Autodesk Fusion 360 part; units mm, degrees
note: some values were not read from the file. Set by a fixed rule: which sketch regions a step uses.
(part 14 of 59)
  spline S77 degree 5 poles (17.8091, 35.4448) (17.8092, 35.4448) (17.8093, 35.445) (17.8095, 35.4453) (17.8098, 35.4457) (17.8103, 35.4463) (17.8108, 35.4469) (17.8114, 35.4477) (17.812, 35.4486) (17.8127, 35.4496) (17.8135, 35.4506) (17.8144, 35.4518) (17.8153, 35.453) (17.8162, 35.4543) (17.8172, 35.4557) (17.8183, 35.4572) (17.8195, 35.4588) (17.8207, 35.4604) (17.8219, 35.4622) (17.8232, 35.464) (17.8246, 35.4659) (17.826, 35.4679) (17.8274, 35.4699) (17.8289, 35.4721) (17.8305, 35.4743) (17.8321, 35.4766) (17.8337, 35.479) (17.8354, 35.4814) (17.8372, 35.484) (17.8389, 35.4866) (17.8408, 35.4893) (17.8427, 35.492) (17.8446, 35.4948) (17.8465, 35.4978) (17.8485, 35.5007) (17.8506, 35.5038) (17.8527, 35.5069) (17.8548, 35.5101) (17.857, 35.5134) (17.8592, 35.5167) (17.8614, 35.5201) (17.8637, 35.5236) (17.866, 35.5271) (17.8683, 35.5308) (17.8707, 35.5344) (17.8731, 35.5382) (17.8756, 35.542) (17.8781, 35.5459) (17.8806, 35.5499) (17.8831, 35.5539) (17.8857, 35.558) (17.8883, 35.5621) (17.891, 35.5664) (17.8937, 35.5706) (17.8964, 35.575) (17.8991, 35.5794) (17.9019, 35.5839) (17.9047, 35.5884) (17.9075, 35.593) (17.9103, 35.5977) (17.9132, 35.6024) (17.9161, 35.6072) (17.9191, 35.6121) (17.922, 35.617) (17.925, 35.622) (17.928, 35.627) (17.931, 35.6321) (17.9341, 35.6373) (17.9372, 35.6425) (17.9403, 35.6478) (17.9434, 35.6531) (17.9466, 35.6585) (17.9497, 35.664) (17.9529, 35.6695) (17.9562, 35.6751) (17.9594, 35.6807) (17.9627, 35.6864) (17.9659, 35.6921) (17.9692, 35.6979) (17.9726, 35.7038) (17.9759, 35.7097) (17.9793, 35.7157) (17.9826, 35.7217) (17.986, 35.7278) (17.9895, 35.734) (17.9929, 35.7402) (17.9963, 35.7464) (17.9998, 35.7527) (18.0033, 35.7591) (18.0068, 35.7655) (18.0103, 35.772) (18.0139, 35.7785) (18.0174, 35.7851) (18.021, 35.7918) (18.0246, 35.7984) (18.0282, 35.8052) (18.0318, 35.812) (18.0354, 35.8188) (18.039, 35.8257) (18.0427, 35.8327) (18.0464, 35.8397) (18.0501, 35.8468) (18.0538, 35.8539) (18.0575, 35.861) (18.0612, 35.8683) (18.0649, 35.8755) (18.0687, 35.8828) (18.0724, 35.8902) (18.0762, 35.8976) (18.08, 35.9051) (18.0838, 35.9126) (18.0876, 35.9202) (18.0914, 35.9278) (18.0952, 35.9355) (18.0991, 35.9432) (18.1029, 35.951) (18.1068, 35.9588) (18.1106, 35.9666) (18.1145, 35.9746) (18.1184, 35.9825) (18.1223, 35.9905) (18.1262, 35.9986) (18.1301, 36.0067) (18.134, 36.0149) (18.1379, 36.0231) (18.1419, 36.0313) (18.1458, 36.0396) (18.1498, 36.048) (18.1537, 36.0564) (18.1577, 36.0648) (18.1617, 36.0733) (18.1657, 36.0818) (18.1696, 36.0904) (18.1736, 36.0991) (18.1776, 36.1077) (18.1816, 36.1165) (18.1857, 36.1252) (18.1897, 36.134) (18.1937, 36.1429) (18.1977, 36.1518) (18.2018, 36.1607) (18.2058, 36.1697) (18.2098, 36.1788) (18.2139, 36.1879) (18.2179, 36.197) (18.222, 36.2062) (18.226, 36.2154) (18.2301, 36.2247) (18.2342, 36.234) (18.2383, 36.2433) (18.2423, 36.2527) (18.2464, 36.2622) (18.2505, 36.2716) (18.2546, 36.2812) (18.2587, 36.2907) (18.2627, 36.3004) (18.2668, 36.31) (18.2709, 36.3197) (18.275, 36.3295) (18.2791, 36.3393) (18.2832, 36.3491) (18.2873, 36.359) (18.2914, 36.3689) (18.2955, 36.3788) (18.2996, 36.3888) (18.3038, 36.3989) (18.3079, 36.409) (18.312, 36.4191) (18.3161, 36.4292) (18.3202, 36.4395) (18.3243, 36.4497) (18.3284, 36.46) (18.3325, 36.4703) (18.3366, 36.4807) (18.3408, 36.4911) (18.3449, 36.5016) (18.349, 36.5121) (18.3531, 36.5226) (18.3572, 36.5332) (18.3613, 36.5438) (18.3654, 36.5545) (18.3695, 36.5652) (18.3736, 36.5759) (18.3777, 36.5867) (18.3818, 36.5975) (18.3859, 36.6084) (18.39, 36.6193) (18.3941, 36.6302) (18.3982, 36.6412) (18.4023, 36.6522) (18.4064, 36.6633) (18.4105, 36.6744) (18.4146, 36.6855) (18.4187, 36.6967) (18.4228, 36.7079) (18.4269, 36.7191) (18.4309, 36.7304) (18.435, 36.7417) (18.4391, 36.7531) (18.4431, 36.7645) (18.4472, 36.776) (18.4513, 36.7874) (18.4553, 36.799) (18.4594, 36.8105) (18.4634, 36.8221) (18.4675, 36.8337) (18.4715, 36.8454) (18.4756, 36.8571) (18.4796, 36.8689) (18.4836, 36.8806) (18.4877, 36.8925) (18.4917, 36.9043) (18.4957, 36.9162) (18.4997, 36.9281) (18.5037, 36.9401) (18.5077, 36.9521) (18.5117, 36.9642) (18.5157, 36.9762) (18.5197, 36.9884) (18.5237, 37.0005) (18.5277, 37.0127) (18.5316, 37.0249) (18.5356, 37.0372) (18.5395, 37.0495) (18.5435, 37.0618) (18.5475, 37.0742) (18.5514, 37.0866) (18.5553, 37.099) (18.5593, 37.1115) (18.5632, 37.124) (18.5671, 37.1365) (18.571, 37.1491) (18.5749, 37.1617) (18.5788, 37.1744) (18.5827, 37.1871) (18.5866, 37.1998) (18.5905, 37.2125) (18.5943, 37.2253) (18.5982, 37.2382) (18.6021, 37.251) (18.6059, 37.2639) (18.609, 37.2743) (18.6113, 37.282) (18.6128, 37.2872) (18.6136, 37.2898) knots 0 0 0 0 0 0 0.00416667 0.00833333 0.0125 0.01666667 0.02083333 0.025 0.02916667 0.03333333 0.0375 0.04166667 0.04583333 0.05 0.05416667 0.05833333 0.0625 0.06666667 0.07083333 0.075 0.07916667 0.08333333 0.0875 0.09166667 0.09583333 0.1 0.10416667 0.10833333 0.1125 0.11666667 0.12083333 0.125 0.12916667 0.13333333 0.1375 0.14166667 0.14583333 0.15 0.15416667 0.15833333 0.1625 0.16666667 0.17083333 0.175 0.17916667 0.18333333 0.1875 0.19166667 0.19583333 0.2 0.20416667 0.20833333 0.2125 0.21666667 0.22083333 0.225 0.22916667 0.23333333 0.2375 0.24166667 0.24583333 0.25 0.25416667 0.25833333 0.2625 0.26666667 0.27083333 0.275 0.27916667 0.28333333 0.2875 0.29166667 0.29583333 0.3 0.30416667 0.30833333 0.3125 0.31666667 0.32083333 0.325 0.32916667 0.33333333 0.3375 0.34166667 0.34583333 0.35 0.35416667 0.35833333 0.3625 0.36666667 0.37083333 0.375 0.37916667 0.38333333 0.3875 0.39166667 0.39583333 0.4 0.40416667 0.40833333 0.4125 0.41666667 0.42083333 0.425 0.42916667 0.43333333 0.4375 0.44166667 0.44583333 0.45 0.45416667 0.45833333 0.4625 0.46666667 0.47083333 0.475 0.47916667 0.48333333 0.4875 0.49166667 0.49583333 0.5 0.50416667 0.50833333 0.5125 0.51666667 0.52083333 0.525 0.52916667 0.53333333 0.5375 0.54166667 0.54583333 0.55 0.55416667 0.55833333 0.5625 0.56666667 0.57083333 0.575 0.57916667 0.58333333 0.5875 0.59166667 0.59583333 0.6 0.60416667 0.60833333 0.6125 0.61666667 0.62083333 0.625 0.62916667 0.63333333 0.6375 0.64166667 0.64583333 0.65 0.65416667 0.65833333 0.6625 0.66666667 0.67083333 0.675 0.67916667 0.68333333 0.6875 0.69166667 0.69583333 0.7 0.70416667 0.70833333 0.7125 0.71666667 0.72083333 0.725 0.72916667 0.73333333 0.7375 0.74166667 0.74583333 0.75 0.75416667 0.75833333 0.7625 0.76666667 0.77083333 0.775 0.77916667 0.78333333 0.7875 0.79166667 0.79583333 0.8 0.80416667 0.80833333 0.8125 0.81666667 0.82083333 0.825 0.82916667 0.83333333 0.8375 0.84166667 0.84583333 0.85 0.85416667 0.85833333 0.8625 0.86666667 0.87083333 0.875 0.87916667 0.88333333 0.8875 0.89166667 0.89583333 0.9 0.90416667 0.90833333 0.9125 0.91666667 0.92083333 0.925 0.92916667 0.93333333 0.9375 0.94166667 0.94583333 0.95 0.95416667 0.95833333 0.9625 0.96666667 0.97083333 0.975 0.97916667 0.98333333 0.9875 0.99166667 0.99583333 1 1 1 1 1 1
  arc A85 (25.3417, -1.078) -> (25.8803, -0.0209) centre (0, 12.5) ccw
  spline S78 degree 5 poles (3.9508, 41.2753) (3.9508, 41.2754) (3.9508, 41.2756) (3.9509, 41.2759) (3.9509, 41.2764) (3.951, 41.2772) (3.9511, 41.278) (3.9512, 41.279) (3.9514, 41.2801) (3.9515, 41.2813) (3.9517, 41.2826) (3.9518, 41.284) (3.952, 41.2855) (3.9522, 41.2871) (3.9523, 41.2889) (3.9525, 41.2907) (3.9527, 41.2926) (3.9529, 41.2946) (3.9531, 41.2968) (3.9534, 41.299) (3.9536, 41.3013) (3.9538, 41.3037) (3.954, 41.3063) (3.9543, 41.3089) (3.9545, 41.3116) (3.9547, 41.3144) (3.955, 41.3172) (3.9552, 41.3202) (3.9555, 41.3233) (3.9557, 41.3264) (3.9559, 41.3297) (3.9562, 41.333) (3.9564, 41.3364) (3.9567, 41.3399) (3.9569, 41.3435) (3.9572, 41.3472) (3.9574, 41.3509) (3.9577, 41.3547) (3.9579, 41.3586) (3.9581, 41.3626) (3.9584, 41.3667) (3.9586, 41.3709) (3.9588, 41.3751) (3.959, 41.3794) (3.9593, 41.3838) (3.9595, 41.3882) (3.9597, 41.3928) (3.9599, 41.3974) (3.9601, 41.4021) (3.9603, 41.4068) (3.9605, 41.4117) (3.9607, 41.4166) (3.9609, 41.4215) (3.961, 41.4266) (3.9612, 41.4317) (3.9614, 41.4369) (3.9615, 41.4422) (3.9617, 41.4475) (3.9618, 41.4529) (3.962, 41.4584) (3.9621, 41.4639) (3.9622, 41.4695) (3.9623, 41.4752) (3.9624, 41.4809) (3.9625, 41.4867) (3.9626, 41.4926) (3.9627, 41.4985) (3.9627, 41.5045) (3.9628, 41.5106) (3.9629, 41.5167) (3.9629, 41.5229) (3.9629, 41.5291) (3.9629, 41.5355) (3.963, 41.5418) (3.963, 41.5483) (3.9629, 41.5548) (3.9629, 41.5613) (3.9629, 41.568) (3.9628, 41.5746) (3.9628, 41.5814) (3.9627, 41.5882) (3.9626, 41.595) (3.9626, 41.6019) (3.9625, 41.6089) (3.9623, 41.6159) (3.9622, 41.623) (3.9621, 41.6302) (3.9619, 41.6374) (3.9618, 41.6446) (3.9616, 41.6519) (3.9614, 41.6593) (3.9612, 41.6667) (3.961, 41.6742) (3.9607, 41.6817) (3.9605, 41.6893) (3.9603, 41.697) (3.96, 41.7047) (3.9597, 41.7124) (3.9594, 41.7202) (3.9591, 41.7281) (3.9588, 41.736) (3.9584, 41.7439) (3.9581, 41.7519) (3.9577, 41.76) (3.9573, 41.7681) (3.9569, 41.7763) (3.9565, 41.7845) (3.9561, 41.7927) (3.9556, 41.801) (3.9552, 41.8094) (3.9547, 41.8178) (3.9542, 41.8263) (3.9537, 41.8348) (3.9532, 41.8433) (3.9526, 41.8519) (3.9521, 41.8606) (3.9515, 41.8693) (3.9509, 41.878) (3.9503, 41.8868) (3.9497, 41.8957) (3.9491, 41.9045) (3.9484, 41.9135) (3.9478, 41.9225) (3.9471, 41.9315) (3.9464, 41.9406) (3.9457, 41.9497) (3.9449, 41.9588) (3.9442, 41.968) (3.9434, 41.9773) (3.9426, 41.9866) (3.9418, 41.9959) (3.941, 42.0053) (3.9402, 42.0147) (3.9393, 42.0242) (3.9384, 42.0337) (3.9375, 42.0433) (3.9366, 42.0529) (3.9357, 42.0625) (3.9348, 42.0722) (3.9338, 42.0819) (3.9328, 42.0917) (3.9318, 42.1015) (3.9308, 42.1113) (3.9297, 42.1212) (3.9287, 42.1312) (3.9276, 42.1411) (3.9265, 42.1512) (3.9254, 42.1612) (3.9243, 42.1713) (3.9231, 42.1814) (3.922, 42.1916) (3.9208, 42.2018) (3.9196, 42.2121) (3.9183, 42.2224) (3.9171, 42.2327) (3.9158, 42.2431) (3.9145, 42.2535) (3.9132, 42.264) (3.9119, 42.2744) (3.9106, 42.285) (3.9092, 42.2955) (3.9078, 42.3061) (3.9064, 42.3168) (3.905, 42.3274) (3.9035, 42.3382) (3.9021, 42.3489) (3.9006, 42.3597) (3.8991, 42.3705) (3.8976, 42.3814) (3.896, 42.3923) (3.8945, 42.4032) (3.8929, 42.4142) (3.8913, 42.4252) (3.8896, 42.4362) (3.888, 42.4473) (3.8863, 42.4584) (3.8846, 42.4696) (3.8829, 42.4807) (3.8812, 42.492) (3.8795, 42.5032) (3.8777, 42.5145) (3.8759, 42.5258) (3.8741, 42.5372) (3.8722, 42.5486) (3.8704, 42.56) (3.8685, 42.5714) (3.8666, 42.5829) (3.8647, 42.5944) (3.8628, 42.606) (3.8608, 42.6176) (3.8588, 42.6292) (3.8568, 42.6409) (3.8548, 42.6525) (3.8527, 42.6643) (3.8507, 42.676) (3.8486, 42.6878) (3.8464, 42.6996) (3.8443, 42.7115) (3.8422, 42.7233) (3.84, 42.7353) (3.8378, 42.7472) (3.8356, 42.7592) (3.8333, 42.7712) (3.831, 42.7832) (3.8288, 42.7953) (3.8264, 42.8074) (3.8241, 42.8195) (3.8217, 42.8317) (3.8194, 42.8439) (3.817, 42.8561) (3.8145, 42.8683) (3.8121, 42.8806) (3.8096, 42.8929) (3.8071, 42.9053) (3.8046, 42.9176) (3.8021, 42.93) (3.7995, 42.9424) (3.797, 42.9549) (3.7943, 42.9674) (3.7917, 42.9799) (3.7891, 42.9924) (3.7864, 43.005) (3.7837, 43.0176) (3.781, 43.0302) (3.7782, 43.0429) (3.7755, 43.0556) (3.7727, 43.0683) (3.7699, 43.081) (3.767, 43.0938) (3.7642, 43.1066) (3.7613, 43.1194) (3.7584, 43.1323) (3.7555, 43.1451) (3.7525, 43.158) (3.7496, 43.171) (3.7466, 43.1839) (3.7435, 43.1969) (3.7405, 43.2099) (3.7374, 43.223) (3.7343, 43.236) (3.7312, 43.2491) (3.7287, 43.2596) (3.7268, 43.2675) (3.7256, 43.2728) (3.7249, 43.2754) knots 0 0 0 0 0 0 0.00416667 0.00833333 0.0125 0.01666667 0.02083333 0.025 0.02916667 0.03333333 0.0375 0.04166667 0.04583333 0.05 0.05416667 0.05833333 0.0625 0.06666667 0.07083333 0.075 0.07916667 0.08333333 0.0875 0.09166667 0.09583333 0.1 0.10416667 0.10833333 0.1125 0.11666667 0.12083333 0.125 0.12916667 0.13333333 0.1375 0.14166667 0.14583333 0.15 0.15416667 0.15833333 0.1625 0.16666667 0.17083333 0.175 0.17916667 0.18333333 0.1875 0.19166667 0.19583333 0.2 0.20416667 0.20833333 0.2125 0.21666667 0.22083333 0.225 0.22916667 0.23333333 0.2375 0.24166667 0.24583333 0.25 0.25416667 0.25833333 0.2625 0.26666667 0.27083333 0.275 0.27916667 0.28333333 0.2875 0.29166667 0.29583333 0.3 0.30416667 0.30833333 0.3125 0.31666667 0.32083333 0.325 0.32916667 0.33333333 0.3375 0.34166667 0.34583333 0.35 0.35416667 0.35833333 0.3625 0.36666667 0.37083333 0.375 0.37916667 0.38333333 0.3875 0.39166667 0.39583333 0.4 0.40416667 0.40833333 0.4125 0.41666667 0.42083333 0.425 0.42916667 0.43333333 0.4375 0.44166667 0.44583333 0.45 0.45416667 0.45833333 0.4625 0.46666667 0.47083333 0.475 0.47916667 0.48333333 0.4875 0.49166667 0.49583333 0.5 0.50416667 0.50833333 0.5125 0.51666667 0.52083333 0.525 0.52916667 0.53333333 0.5375 0.54166667 0.54583333 0.55 0.55416667 0.55833333 0.5625 0.56666667 0.57083333 0.575 0.57916667 0.58333333 0.5875 0.59166667 0.59583333 0.6 0.60416667 0.60833333 0.6125 0.61666667 0.62083333 0.625 0.62916667 0.63333333 0.6375 0.64166667 0.64583333 0.65 0.65416667 0.65833333 0.6625 0.66666667 0.67083333 0.675 0.67916667 0.68333333 0.6875 0.69166667 0.69583333 0.7 0.70416667 0.70833333 0.7125 0.71666667 0.72083333 0.725 0.72916667 0.73333333 0.7375 0.74166667 0.74583333 0.75 0.75416667 0.75833333 0.7625 0.76666667 0.77083333 0.775 0.77916667 0.78333333 0.7875 0.79166667 0.79583333 0.8 0.80416667 0.80833333 0.8125 0.81666667 0.82083333 0.825 0.82916667 0.83333333 0.8375 0.84166667 0.84583333 0.85 0.85416667 0.85833333 0.8625 0.86666667 0.87083333 0.875 0.87916667 0.88333333 0.8875 0.89166667 0.89583333 0.9 0.90416667 0.90833333 0.9125 0.91666667 0.92083333 0.925 0.92916667 0.93333333 0.9375 0.94166667 0.94583333 0.95 0.95416667 0.95833333 0.9625 0.96666667 0.97083333 0.975 0.97916667 0.98333333 0.9875 0.99166667 0.99583333 1 1 1 1 1 1
  line L159 (28.7355, 11.5881) -> (29.0298, 11.5787)
  line L160 (0.9213, -16.5307) -> (0.9213, -16.5298)
  line L161 (28.7745, 8.5493) -> (28.7753, 8.5492)
  line L162 (2.1182, -16.4671) -> (2.1183, -16.4679)
  arc A86 (28.6734, 10.4033) -> (28.7355, 11.5881) centre (0, 12.5) ccw
  line L163 (28.9671, 10.3818) -> (28.6734, 10.4033)
  line L164 (-8.0948, -15.3945) -> (-8.0945, -15.3937)
  line L165 (-6.8665, -15.418) -> (-6.9368, -15.7039)
  arc A87 (30.7754, 8.7751) -> (30.8773, 9.745) centre (0, 12.5) ccw
  line L166 (0.9213, -16.5298) -> (0.9119, -16.2355)
  spline S79 degree 5 poles (30.7754, 16.2249) (30.7728, 16.2256) (30.7675, 16.2268) (30.7596, 16.2287) (30.7491, 16.2312) (30.736, 16.2343) (30.723, 16.2374) (30.7099, 16.2405) (30.6969, 16.2435) (30.6839, 16.2466) (30.671, 16.2496) (30.658, 16.2525) (30.6451, 16.2555) (30.6323, 16.2584) (30.6194, 16.2613) (30.6066, 16.2642) (30.5938, 16.267) (30.581, 16.2699) (30.5683, 16.2727) (30.5556, 16.2755) (30.5429, 16.2782) (30.5302, 16.281) (30.5176, 16.2837) (30.505, 16.2864) (30.4924, 16.2891) (30.4799, 16.2917) (30.4674, 16.2943) (30.4549, 16.297) (30.4424, 16.2995) (30.43, 16.3021) (30.4176, 16.3046) (30.4053, 16.3071) (30.3929, 16.3096) (30.3806, 16.3121) (30.3683, 16.3145) (30.3561, 16.317) (30.3439, 16.3194) (30.3317, 16.3217) (30.3195, 16.3241) (30.3074, 16.3264) (30.2953, 16.3288) (30.2832, 16.331) (30.2712, 16.3333) (30.2592, 16.3356) (30.2472, 16.3378) (30.2353, 16.34) (30.2233, 16.3422) (30.2115, 16.3443) (30.1996, 16.3464) (30.1878, 16.3486) (30.176, 16.3507) (30.1643, 16.3527) (30.1525, 16.3548) (30.1409, 16.3568) (30.1292, 16.3588) (30.1176, 16.3608) (30.106, 16.3628) (30.0944, 16.3647) (30.0829, 16.3666) (30.0714, 16.3685) (30.06, 16.3704) (30.0486, 16.3722) (30.0372, 16.3741) (30.0258, 16.3759) (30.0145, 16.3777) (30.0032, 16.3795) (29.992, 16.3812) (29.9807, 16.3829) (29.9696, 16.3846) (29.9584, 16.3863) (29.9473, 16.388) (29.9362, 16.3896) (29.9252, 16.3913) (29.9142, 16.3929) (29.9032, 16.3945) (29.8923, 16.396) (29.8814, 16.3976) (29.8705, 16.3991) (29.8597, 16.4006) (29.8489, 16.4021) (29.8382, 16.4035) (29.8274, 16.405) (29.8168, 16.4064) (29.8061, 16.4078) (29.7955, 16.4092) (29.785, 16.4106) (29.7744, 16.4119) (29.764, 16.4132) (29.7535, 16.4145) (29.7431, 16.4158) (29.7327, 16.4171) (29.7224, 16.4183) (29.7121, 16.4196) (29.7018, 16.4208) (29.6916, 16.422) (29.6814, 16.4231) (29.6713, 16.4243) (29.6612, 16.4254) (29.6512, 16.4265) (29.6411, 16.4276) (29.6312, 16.4287) (29.6212, 16.4297) (29.6113, 16.4308) (29.6015, 16.4318) (29.5917, 16.4328) (29.5819, 16.4338) (29.5722, 16.4348) (29.5625, 16.4357) (29.5529, 16.4366) (29.5433, 16.4375) (29.5337, 16.4384) (29.5242, 16.4393) (29.5147, 16.4402) (29.5053, 16.441) (29.4959, 16.4418) (29.4866, 16.4426) (29.4773, 16.4434) (29.468, 16.4442) (29.4588, 16.4449) (29.4497, 16.4457) (29.4406, 16.4464) (29.4315, 16.4471) (29.4225, 16.4478) (29.4135, 16.4484) (29.4045, 16.4491) (29.3957, 16.4497) (29.3868, 16.4503) (29.378, 16.4509) (29.3693, 16.4515) (29.3606, 16.4521) (29.3519, 16.4526) (29.3433, 16.4532) (29.3348, 16.4537) (29.3263, 16.4542) (29.3178, 16.4547) (29.3094, 16.4552) (29.301, 16.4556) (29.2927, 16.4561) (29.2845, 16.4565) (29.2763, 16.4569) (29.2681, 16.4573) (29.26, 16.4577) (29.2519, 16.4581) (29.2439, 16.4584) (29.236, 16.4588) (29.2281, 16.4591) (29.2202, 16.4594) (29.2124, 16.4597) (29.2047, 16.46) (29.197, 16.4603) (29.1893, 16.4605) (29.1817, 16.4607) (29.1742, 16.461) (29.1667, 16.4612) (29.1593, 16.4614) (29.1519, 16.4616) (29.1446, 16.4618) (29.1374, 16.4619) (29.1302, 16.4621) (29.123, 16.4622) (29.1159, 16.4623) (29.1089, 16.4625) (29.1019, 16.4626) (29.095, 16.4626) (29.0882, 16.4627) (29.0814, 16.4628) (29.0746, 16.4628) (29.068, 16.4629) (29.0613, 16.4629) (29.0548, 16.4629) (29.0483, 16.463) (29.0418, 16.463) (29.0355, 16.4629) (29.0291, 16.4629) (29.0229, 16.4629) (29.0167, 16.4629) (29.0106, 16.4628) (29.0045, 16.4627) (28.9985, 16.4627) (28.9926, 16.4626) (28.9867, 16.4625) (28.9809, 16.4624) (28.9752, 16.4623) (28.9695, 16.4622) (28.9639, 16.4621) (28.9584, 16.462) (28.9529, 16.4618) (28.9475, 16.4617) (28.9422, 16.4615) (28.9369, 16.4614) (28.9317, 16.4612) (28.9266, 16.461) (28.9215, 16.4609) (28.9166, 16.4607) (28.9117, 16.4605) (28.9068, 16.4603) (28.9021, 16.4601) (28.8974, 16.4599) (28.8928, 16.4597) (28.8882, 16.4595) (28.8838, 16.4593) (28.8794, 16.459) (28.8751, 16.4588) (28.8709, 16.4586) (28.8667, 16.4584) (28.8626, 16.4581) (28.8586, 16.4579) (28.8547, 16.4577) (28.8509, 16.4574) (28.8472, 16.4572) (28.8435, 16.4569) (28.8399, 16.4567) (28.8364, 16.4564) (28.833, 16.4562) (28.8297, 16.4559) (28.8264, 16.4557) (28.8233, 16.4555) (28.8202, 16.4552) (28.8172, 16.455) (28.8144, 16.4547) (28.8116, 16.4545) (28.8089, 16.4543) (28.8063, 16.454) (28.8037, 16.4538) (28.8013, 16.4536) (28.799, 16.4534) (28.7968, 16.4531) (28.7946, 16.4529) (28.7926, 16.4527) (28.7907, 16.4525) (28.7889, 16.4523) (28.7871, 16.4522) (28.7855, 16.452) (28.784, 16.4518) (28.7826, 16.4517) (28.7813, 16.4515) (28.7801, 16.4514) (28.779, 16.4512) (28.778, 16.4511) (28.7772, 16.451) (28.7764, 16.4509) (28.7759, 16.4509) (28.7756, 16.4508) (28.7754, 16.4508) (28.7753, 16.4508) knots -1 -1 -1 -1 -1 -1 -0.99583333 -0.99166667 -0.9875 -0.98333333 -0.97916667 -0.975 -0.97083333 -0.96666667 -0.9625 -0.95833333 -0.95416667 -0.95 -0.94583333 -0.94166667 -0.9375 -0.93333333 -0.92916667 -0.925 -0.92083333 -0.91666667 -0.9125 -0.90833333 -0.90416667 -0.9 -0.89583333 -0.89166667 -0.8875 -0.88333333 -0.87916667 -0.875 -0.87083333 -0.86666667 -0.8625 -0.85833333 -0.85416667 -0.85 -0.84583333 -0.84166667 -0.8375 -0.83333333 -0.82916667 -0.825 -0.82083333 -0.81666667 -0.8125 -0.80833333 -0.80416667 -0.8 -0.79583333 -0.79166667 -0.7875 -0.78333333 -0.77916667 -0.775 -0.77083333 -0.76666667 -0.7625 -0.75833333 -0.75416667 -0.75 -0.74583333 -0.74166667 -0.7375 -0.73333333 -0.72916667 -0.725 -0.72083333 -0.71666667 -0.7125 -0.70833333 -0.70416667 -0.7 -0.69583333 -0.69166667 -0.6875 -0.68333333 -0.67916667 -0.675 -0.67083333 -0.66666667 -0.6625 -0.65833333 -0.65416667 -0.65 -0.64583333 -0.64166667 -0.6375 -0.63333333 -0.62916667 -0.625 -0.62083333 -0.61666667 -0.6125 -0.60833333 -0.60416667 -0.6 -0.59583333 -0.59166667 -0.5875 -0.58333333 -0.57916667 -0.575 -0.57083333 -0.56666667 -0.5625 -0.55833333 -0.55416667 -0.55 -0.54583333 -0.54166667 -0.5375 -0.53333333 -0.52916667 -0.525 -0.52083333 -0.51666667 -0.5125 -0.50833333 -0.50416667 -0.5 -0.49583333 -0.49166667 -0.4875 -0.48333333 -0.47916667 -0.475 -0.47083333 -0.46666667 -0.4625 -0.45833333 -0.45416667 -0.45 -0.44583333 -0.44166667 -0.4375 -0.43333333 -0.42916667 -0.425 -0.42083333 -0.41666667 -0.4125 -0.40833333 -0.40416667 -0.4 -0.39583333 -0.39166667 -0.3875 -0.38333333 -0.37916667 -0.375 -0.37083333 -0.36666667 -0.3625 -0.35833333 -0.35416667 -0.35 -0.34583333 -0.34166667 -0.3375 -0.33333333 -0.32916667 -0.325 -0.32083333 -0.31666667 -0.3125 -0.30833333 -0.30416667 -0.3 -0.29583333 -0.29166667 -0.2875 -0.28333333 -0.27916667 -0.275 -0.27083333 -0.26666667 -0.2625 -0.25833333 -0.25416667 -0.25 -0.24583333 -0.24166667 -0.2375 -0.23333333 -0.22916667 -0.225 -0.22083333 -0.21666667 -0.2125 -0.20833333 -0.20416667 -0.2 -0.19583333 -0.19166667 -0.1875 -0.18333333 -0.17916667 -0.175 -0.17083333 -0.16666667 -0.1625 -0.15833333 -0.15416667 -0.15 -0.14583333 -0.14166667 -0.1375 -0.13333333 -0.12916667 -0.125 -0.12083333 -0.11666667 -0.1125 -0.10833333 -0.10416667 -0.1 -0.09583333 -0.09166667 -0.0875 -0.08333333 -0.07916667 -0.075 -0.07083333 -0.06666667 -0.0625 -0.05833333 -0.05416667 -0.05 -0.04583333 -0.04166667 -0.0375 -0.03333333 -0.02916667 -0.025 -0.02083333 -0.01666667 -0.0125 -0.00833333 -0.00416667 0 0 0 0 0 0
  line L167 (28.4828, 8.5894) -> (28.7745, 8.5493)
  line L168 (27.3243, 2.6531) -> (27.3251, 2.6528)
  line L169 (3.9508, -16.2753) -> (3.9507, -16.2745)
  spline S80 degree 5 poles (-0.9213, -16.5307) (-0.9213, -16.5307) (-0.9213, -16.5309) (-0.9213, -16.5313) (-0.9213, -16.5318) (-0.9213, -16.5325) (-0.9213, -16.5334) (-0.9214, -16.5344) (-0.9214, -16.5355) (-0.9214, -16.5367) (-0.9214, -16.538) (-0.9214, -16.5394) (-0.9214, -16.5409) (-0.9214, -16.5425) (-0.9214, -16.5443) (-0.9214, -16.5461) (-0.9214, -16.5481) (-0.9214, -16.5501) (-0.9214, -16.5522) (-0.9214, -16.5545) (-0.9214, -16.5568) (-0.9213, -16.5592) (-0.9213, -16.5618) (-0.9212, -16.5644) (-0.9212, -16.5671) (-0.9211, -16.5699) (-0.9211, -16.5728) (-0.921, -16.5758) (-0.9209, -16.5788) (-0.9208, -16.582) (-0.9208, -16.5852) (-0.9206, -16.5886) (-0.9205, -16.592) (-0.9204, -16.5955) (-0.9203, -16.5991) (-0.9201, -16.6028) (-0.92, -16.6065) (-0.9198, -16.6103) (-0.9197, -16.6143) (-0.9195, -16.6183) (-0.9193, -16.6223) (-0.9191, -16.6265) (-0.9189, -16.6307) (-0.9186, -16.635) (-0.9184, -16.6394) (-0.9182, -16.6439) (-0.9179, -16.6484) (-0.9176, -16.653) (-0.9173, -16.6577) (-0.917, -16.6624) (-0.9167, -16.6673) (-0.9164, -16.6722) (-0.9161, -16.6771) (-0.9157, -16.6822) (-0.9153, -16.6873) (-0.915, -16.6925) (-0.9146, -16.6977) (-0.9141, -16.703) (-0.9137, -16.7084) (-0.9133, -16.7139) (-0.9128, -16.7194) (-0.9124, -16.725) (-0.9119, -16.7306) (-0.9114, -16.7363) (-0.9109, -16.7421) (-0.9103, -16.748) (-0.9098, -16.7539) (-0.9092, -16.7599) (-0.9087, -16.7659) (-0.9081, -16.772) (-0.9075, -16.7781) (-0.9068, -16.7844) (-0.9062, -16.7906) (-0.9055, -16.797) (-0.9049, -16.8034) (-0.9042, -16.8099) (-0.9035, -16.8164) (-0.9027, -16.823) (-0.902, -16.8296) (-0.9012, -16.8363) (-0.9005, -16.843) (-0.8997, -16.8498) (-0.8989, -16.8567) (-0.898, -16.8636) (-0.8972, -16.8706) (-0.8963, -16.8777) (-0.8954, -16.8847) (-0.8945, -16.8919) (-0.8936, -16.8991) (-0.8927, -16.9063) (-0.8917, -16.9137) (-0.8907, -16.921) (-0.8897, -16.9284) (-0.8887, -16.9359) (-0.8877, -16.9434) (-0.8866, -16.951) (-0.8856, -16.9586) (-0.8845, -16.9663) (-0.8834, -16.974) (-0.8822, -16.9818) (-0.8811, -16.9896) (-0.8799, -16.9975) (-0.8787, -17.0054) (-0.8775, -17.0134) (-0.8763, -17.0214) (-0.875, -17.0295) (-0.8738, -17.0376) (-0.8725, -17.0458) (-0.8712, -17.054) (-0.8698, -17.0623) (-0.8685, -17.0706) (-0.8671, -17.0789) (-0.8657, -17.0873) (-0.8643, -17.0958) (-0.8629, -17.1043) (-0.8614, -17.1128) (-0.86, -17.1214) (-0.8585, -17.1301) (-0.8569, -17.1388) (-0.8554, -17.1475) (-0.8538, -17.1563) (-0.8523, -17.1651) (-0.8507, -17.1739) (-0.849, -17.1828) (-0.8474, -17.1918) (-0.8457, -17.2008) (-0.844, -17.2098) (-0.8423, -17.2189) (-0.8406, -17.228) (-0.8388, -17.2372) (-0.8371, -17.2464) (-0.8353, -17.2556) (-0.8334, -17.2649) (-0.8316, -17.2742) (-0.8297, -17.2836) (-0.8279, -17.293) (-0.8259, -17.3025) (-0.824, -17.312) (-0.8221, -17.3215) (-0.8201, -17.3311) (-0.8181, -17.3407) (-0.8161, -17.3503) (-0.814, -17.36) (-0.812, -17.3697) (-0.8099, -17.3795) (-0.8078, -17.3893) (-0.8056, -17.3992) (-0.8035, -17.409) (-0.8013, -17.419) (-0.7991, -17.4289) (-0.7969, -17.4389) (-0.7946, -17.449) (-0.7923, -17.459) (-0.79, -17.4691) (-0.7877, -17.4793) (-0.7854, -17.4895) (-0.783, -17.4997) (-0.7806, -17.5099) (-0.7782, -17.5202) (-0.7758, -17.5306) (-0.7733, -17.5409) (-0.7708, -17.5513) (-0.7683, -17.5618) (-0.7658, -17.5722) (-0.7632, -17.5827) (-0.7606, -17.5933) (-0.758, -17.6038) (-0.7554, -17.6145) (-0.7528, -17.6251) (-0.7501, -17.6358) (-0.7474, -17.6465) (-0.7447, -17.6572) (-0.7419, -17.668) (-0.7391, -17.6788) (-0.7364, -17.6897) (-0.7335, -17.7005) (-0.7307, -17.7114) (-0.7278, -17.7224) (-0.7249, -17.7334) (-0.722, -17.7444) (-0.7191, -17.7554) (-0.7161, -17.7665) (-0.7131, -17.7776) (-0.7101, -17.7887) (-0.7071, -17.7999) (-0.704, -17.8111) (-0.7009, -17.8223) (-0.6978, -17.8336) (-0.6947, -17.8448) (-0.6915, -17.8562) (-0.6883, -17.8675) (-0.6851, -17.8789) (-0.6819, -17.8903) (-0.6786, -17.9017) (-0.6753, -17.9132) (-0.672, -17.9247) (-0.6687, -17.9362) (-0.6653, -17.9478) (-0.6619, -17.9594) (-0.6585, -17.971) (-0.6551, -17.9827) (-0.6516, -17.9943) (-0.6481, -18.006) (-0.6446, -18.0178) (-0.6411, -18.0295) (-0.6375, -18.0413) (-0.6339, -18.0531) (-0.6303, -18.065) (-0.6267, -18.0769) (-0.623, -18.0888) (-0.6193, -18.1007) (-0.6156, -18.1126) (-0.6118, -18.1246) (-0.6081, -18.1366) (-0.6043, -18.1487) (-0.6005, -18.1607) (-0.5966, -18.1728) (-0.5927, -18.185) (-0.5889, -18.1971) (-0.5849, -18.2093) (-0.581, -18.2215) (-0.577, -18.2337) (-0.573, -18.2459) (-0.569, -18.2582) (-0.5649, -18.2705) (-0.5609, -18.2828) (-0.5568, -18.2952) (-0.5526, -18.3076) (-0.5485, -18.32) (-0.5443, -18.3324) (-0.5401, -18.3448) (-0.5359, -18.3573) (-0.5316, -18.3698) (-0.5273, -18.3823) (-0.523, -18.3949) (-0.5187, -18.4075) (-0.5143, -18.4201) (-0.5099, -18.4327) (-0.5055, -18.4453) (-0.5011, -18.458) (-0.4966, -18.4707) (-0.493, -18.4809) (-0.4903, -18.4885) (-0.4885, -18.4936) (-0.4876, -18.4962) knots 0 0 0 0 0 0 0.00416667 0.00833333 0.0125 0.01666667 0.02083333 0.025 0.02916667 0.03333333 0.0375 0.04166667 0.04583333 0.05 0.05416667 0.05833333 0.0625 0.06666667 0.07083333 0.075 0.07916667 0.08333333 0.0875 0.09166667 0.09583333 0.1 0.10416667 0.10833333 0.1125 0.11666667 0.12083333 0.125 0.12916667 0.13333333 0.1375 0.14166667 0.14583333 0.15 0.15416667 0.15833333 0.1625 0.16666667 0.17083333 0.175 0.17916667 0.18333333 0.1875 0.19166667 0.19583333 0.2 0.20416667 0.20833333 0.2125 0.21666667 0.22083333 0.225 0.22916667 0.23333333 0.2375 0.24166667 0.24583333 0.25 0.25416667 0.25833333 0.2625 0.26666667 0.27083333 0.275 0.27916667 0.28333333 0.2875 0.29166667 0.29583333 0.3 0.30416667 0.30833333 0.3125 0.31666667 0.32083333 0.325 0.32916667 0.33333333 0.3375 0.34166667 0.34583333 0.35 0.35416667 0.35833333 0.3625 0.36666667 0.37083333 0.375 0.37916667 0.38333333 0.3875 0.39166667 0.39583333 0.4 0.40416667 0.40833333 0.4125 0.41666667 0.42083333 0.425 0.42916667 0.43333333 0.4375 0.44166667 0.44583333 0.45 0.45416667 0.45833333 0.4625 0.46666667 0.47083333 0.475 0.47916667 0.48333333 0.4875 0.49166667 0.49583333 0.5 0.50416667 0.50833333 0.5125 0.51666667 0.52083333 0.525 0.52916667 0.53333333 0.5375 0.54166667 0.54583333 0.55 0.55416667 0.55833333 0.5625 0.56666667 0.57083333 0.575 0.57916667 0.58333333 0.5875 0.59166667 0.59583333 0.6 0.60416667 0.60833333 0.6125 0.61666667 0.62083333 0.625 0.62916667 0.63333333 0.6375 0.64166667 0.64583333 0.65 0.65416667 0.65833333 0.6625 0.66666667 0.67083333 0.675 0.67916667 0.68333333 0.6875 0.69166667 0.69583333 0.7 0.70416667 0.70833333 0.7125 0.71666667 0.72083333 0.725 0.72916667 0.73333333 0.7375 0.74166667 0.74583333 0.75 0.75416667 0.75833333 0.7625 0.76666667 0.77083333 0.775 0.77916667 0.78333333 0.7875 0.79166667 0.79583333 0.8 0.80416667 0.80833333 0.8125 0.81666667 0.82083333 0.825 0.82916667 0.83333333 0.8375 0.84166667 0.84583333 0.85 0.85416667 0.85833333 0.8625 0.86666667 0.87083333 0.875 0.87916667 0.88333333 0.8875 0.89166667 0.89583333 0.9 0.90416667 0.90833333 0.9125 0.91666667 0.92083333 0.925 0.92916667 0.93333333 0.9375 0.94166667 0.94583333 0.95 0.95416667 0.95833333 0.9625 0.96666667 0.97083333 0.975 0.97916667 0.98333333 0.9875 0.99166667 0.99583333 1 1 1 1 1 1
  spline S81 degree 5 poles (10.9662, -14.3955) (10.9662, -14.3956) (10.9663, -14.3958) (10.9664, -14.3961) (10.9666, -14.3966) (10.9669, -14.3973) (10.9672, -14.3981) (10.9676, -14.399) (10.9681, -14.4) (10.9685, -14.4011) (10.9691, -14.4023) (10.9696, -14.4036) (10.9702, -14.405) (10.9709, -14.4065) (10.9716, -14.408) (10.9724, -14.4097) (10.9731, -14.4115) (10.974, -14.4134) (10.9749, -14.4153) (10.9758, -14.4173) (10.9768, -14.4195) (10.9778, -14.4217) (10.9788, -14.424) (10.9799, -14.4263) (10.9811, -14.4288) (10.9823, -14.4313) (10.9835, -14.4339) (10.9848, -14.4366) (10.9861, -14.4394) (10.9875, -14.4423) (10.9889, -14.4452) (10.9903, -14.4482) (10.9918, -14.4513) (10.9934, -14.4544) (10.9949, -14.4577) (10.9966, -14.461) (10.9982, -14.4643) (10.9999, -14.4678) (11.0017, -14.4713) (11.0035, -14.4748) (11.0053, -14.4785) (11.0072, -14.4822) (11.0091, -14.486) (11.0111, -14.4898) (11.0131, -14.4937) (11.0151, -14.4977) (11.0172, -14.5017) (11.0193, -14.5058) (11.0215, -14.51) (11.0237, -14.5142) (11.0259, -14.5185) (11.0282, -14.5228) (11.0306, -14.5272) (11.0329, -14.5317) (11.0353, -14.5362) (11.0378, -14.5408) (11.0403, -14.5454) (11.0428, -14.5501) (11.0454, -14.5549) (11.048, -14.5597) (11.0507, -14.5645) (11.0534, -14.5694) (11.0561, -14.5744) (11.0589, -14.5794) (11.0617, -14.5845) (11.0646, -14.5896) (11.0675, -14.5948) (11.0704, -14.6) (11.0734, -14.6053) (11.0764, -14.6106) (11.0795, -14.616) (11.0826, -14.6214) (11.0857, -14.6269) (11.0889, -14.6324) (11.0921, -14.638) (11.0954, -14.6436) (11.0987, -14.6493) (11.102, -14.655) (11.1054, -14.6608) (11.1088, -14.6666) (11.1123, -14.6725) (11.1158, -14.6784) (11.1193, -14.6843) (11.1229, -14.6903) (11.1265, -14.6963) (11.1301, -14.7024) (11.1338, -14.7085) (11.1376, -14.7147) (11.1413, -14.7209) (11.1451, -14.7271) (11.149, -14.7334) (11.1529, -14.7397) (11.1568, -14.7461) (11.1608, -14.7525) (11.1648, -14.759) (11.1688, -14.7654) (11.1729, -14.772) (11.177, -14.7785) (11.1812, -14.7851) (11.1854, -14.7918) (11.1896, -14.7985) (11.1939, -14.8052) (11.1982, -14.8119) (11.2025, -14.8187) (11.2069, -14.8256) (11.2113, -14.8324) (11.2158, -14.8393) (11.2203, -14.8463) (11.2248, -14.8533) (11.2294, -14.8603) (11.234, -14.8673) (11.2387, -14.8744) (11.2434, -14.8815) (11.2481, -14.8887) (11.2529, -14.8958) (11.2577, -14.9031) (11.2625, -14.9103) (11.2674, -14.9176) (11.2723, -14.9249) (11.2773, -14.9323) (11.2823, -14.9396) (11.2873, -14.947) (11.2924, -14.9545) (11.2975, -14.962) (11.3026, -14.9695) (11.3078, -14.977) (11.313, -14.9846) (11.3183, -14.9922) (11.3235, -14.9998) (11.3289, -15.0074) (11.3342, -15.0151) (11.3396, -15.0228) (11.3451, -15.0306) (11.3506, -15.0384) (11.3561, -15.0462) (11.3616, -15.054) (11.3672, -15.0618) (11.3728, -15.0697) (11.3785, -15.0776) (11.3842, -15.0856) (11.3899, -15.0936) (11.3957, -15.1015) (11.4015, -15.1096) (11.4074, -15.1176) (11.4132, -15.1257) (11.4192, -15.1338) (11.4251, -15.1419) (11.4311, -15.1501) (11.4371, -15.1582) (11.4432, -15.1665) (11.4493, -15.1747) (11.4554, -15.1829) (11.4616, -15.1912) (11.4678, -15.1995) (11.4741, -15.2078) (11.4803, -15.2162) (11.4867, -15.2246) (11.493, -15.233) (11.4994, -15.2414) (11.5058, -15.2498) (11.5123, -15.2583) (11.5188, -15.2668) (11.5253, -15.2753) (11.5319, -15.2838) (11.5385, -15.2924) (11.5452, -15.301) (11.5518, -15.3096) (11.5585, -15.3182) (11.5653, -15.3268) (11.5721, -15.3355) (11.5789, -15.3442) (11.5858, -15.3529) (11.5927, -15.3616) (11.5996, -15.3704) (11.6065, -15.3791) (11.6135, -15.3879) (11.6206, -15.3967) (11.6276, -15.4055) (11.6348, -15.4144) (11.6419, -15.4233) (11.6491, -15.4322) (11.6563, -15.4411) (11.6635, -15.45) (11.6708, -15.4589) (11.6781, -15.4679) (11.6855, -15.4769) (11.6929, -15.4859) (11.7003, -15.4949) (11.7078, -15.5039) (11.7153, -15.513) (11.7228, -15.5221) (11.7303, -15.5312) (11.7379, -15.5403) (11.7456, -15.5494) (11.7532, -15.5585) (11.7609, -15.5677) (11.7687, -15.5769) (11.7765, -15.5861) (11.7843, -15.5953) (11.7921, -15.6045) (11.8, -15.6137) (11.8079, -15.623) (11.8158, -15.6323) (11.8238, -15.6416) (11.8318, -15.6509) (11.8399, -15.6602) (11.848, -15.6695) (11.8561, -15.6789) (11.8643, -15.6882) (11.8724, -15.6976) (11.8807, -15.707) (11.8889, -15.7164) (11.8972, -15.7259) (11.9055, -15.7353) (11.9139, -15.7447) (11.9223, -15.7542) (11.9307, -15.7637) (11.9392, -15.7732) (11.9477, -15.7827) (11.9562, -15.7922) (11.9648, -15.8018) (11.9734, -15.8113) (11.982, -15.8209) (11.9907, -15.8305) (11.9994, -15.84) (12.0081, -15.8496) (12.0169, -15.8593) (12.0257, -15.8689) (12.0345, -15.8785) (12.0434, -15.8882) (12.0523, -15.8978) (12.0613, -15.9075) (12.0702, -15.9172) (12.0792, -15.9269) (12.0883, -15.9366) (12.0973, -15.9464) (12.1065, -15.9561) (12.1156, -15.9658) (12.1248, -15.9756) (12.134, -15.9854) (12.1432, -15.9951) (12.1506, -16.003) (12.1562, -16.0089) (12.16, -16.0128) (12.1618, -16.0147) knots 0 0 0 0 0 0 0.00416667 0.00833333 0.0125 0.01666667 0.02083333 0.025 0.02916667 0.03333333 0.0375 0.04166667 0.04583333 0.05 0.05416667 0.05833333 0.0625 0.06666667 0.07083333 0.075 0.07916667 0.08333333 0.0875 0.09166667 0.09583333 0.1 0.10416667 0.10833333 0.1125 0.11666667 0.12083333 0.125 0.12916667 0.13333333 0.1375 0.14166667 0.14583333 0.15 0.15416667 0.15833333 0.1625 0.16666667 0.17083333 0.175 0.17916667 0.18333333 0.1875 0.19166667 0.19583333 0.2 0.20416667 0.20833333 0.2125 0.21666667 0.22083333 0.225 0.22916667 0.23333333 0.2375 0.24166667 0.24583333 0.25 0.25416667 0.25833333 0.2625 0.26666667 0.27083333 0.275 0.27916667 0.28333333 0.2875 0.29166667 0.29583333 0.3 0.30416667 0.30833333 0.3125 0.31666667 0.32083333 0.325 0.32916667 0.33333333 0.3375 0.34166667 0.34583333 0.35 0.35416667 0.35833333 0.3625 0.36666667 0.37083333 0.375 0.37916667 0.38333333 0.3875 0.39166667 0.39583333 0.4 0.40416667 0.40833333 0.4125 0.41666667 0.42083333 0.425 0.42916667 0.43333333 0.4375 0.44166667 0.44583333 0.45 0.45416667 0.45833333 0.4625 0.46666667 0.47083333 0.475 0.47916667 0.48333333 0.4875 0.49166667 0.49583333 0.5 0.50416667 0.50833333 0.5125 0.51666667 0.52083333 0.525 0.52916667 0.53333333 0.5375 0.54166667 0.54583333 0.55 0.55416667 0.55833333 0.5625 0.56666667 0.57083333 0.575 0.57916667 0.58333333 0.5875 0.59166667 0.59583333 0.6 0.60416667 0.60833333 0.6125 0.61666667 0.62083333 0.625 0.62916667 0.63333333 0.6375 0.64166667 0.64583333 0.65 0.65416667 0.65833333 0.6625 0.66666667 0.67083333 0.675 0.67916667 0.68333333 0.6875 0.69166667 0.69583333 0.7 0.70416667 0.70833333 0.7125 0.71666667 0.72083333 0.725 0.72916667 0.73333333 0.7375 0.74166667 0.74583333 0.75 0.75416667 0.75833333 0.7625 0.76666667 0.77083333 0.775 0.77916667 0.78333333 0.7875 0.79166667 0.79583333 0.8 0.80416667 0.80833333 0.8125 0.81666667 0.82083333 0.825 0.82916667 0.83333333 0.8375 0.84166667 0.84583333 0.85 0.85416667 0.85833333 0.8625 0.86666667 0.87083333 0.875 0.87916667 0.88333333 0.8875 0.89166667 0.89583333 0.9 0.90416667 0.90833333 0.9125 0.91666667 0.92083333 0.925 0.92916667 0.93333333 0.9375 0.94166667 0.94583333 0.95 0.95416667 0.95833333 0.9625 0.96666667 0.97083333 0.975 0.97916667 0.98333333 0.9875 0.99166667 0.99583333 1 1 1 1 1 1
  line L170 (15.3128, 37.1799) -> (15.3132, 37.1806)
  spline S82 degree 5 poles (28.9679, 14.6183) (28.968, 14.6183) (28.9682, 14.6183) (28.9685, 14.6183) (28.969, 14.6184) (28.9698, 14.6184) (28.9706, 14.6185) (28.9716, 14.6186) (28.9727, 14.6187) (28.9739, 14.6188) (28.9752, 14.6189) (28.9766, 14.6191) (28.9781, 14.6192) (28.9798, 14.6194) (28.9815, 14.6196) (28.9833, 14.6198) (28.9852, 14.62) (28.9873, 14.6202) (28.9894, 14.6204) (28.9916, 14.6207) (28.9939, 14.621) (28.9963, 14.6212) (28.9989, 14.6215) (29.0015, 14.6219) (29.0041, 14.6222) (29.0069, 14.6225) (29.0098, 14.6229) (29.0128, 14.6233) (29.0158, 14.6237) (29.0189, 14.6241) (29.0222, 14.6245) (29.0255, 14.625) (29.0289, 14.6254) (29.0323, 14.6259) (29.0359, 14.6264) (29.0395, 14.627) (29.0432, 14.6275) (29.047, 14.6281) (29.0509, 14.6286) (29.0549, 14.6292) (29.0589, 14.6299) (29.063, 14.6305) (29.0672, 14.6312) (29.0714, 14.6318) (29.0758, 14.6325) (29.0802, 14.6332) (29.0847, 14.634) (29.0892, 14.6347) (29.0938, 14.6355) (29.0985, 14.6363) (29.1033, 14.6371) (29.1081, 14.638) (29.1131, 14.6388) (29.118, 14.6397) (29.1231, 14.6406) (29.1282, 14.6415) (29.1334, 14.6424) (29.1386, 14.6434) (29.1439, 14.6444) (29.1493, 14.6454) (29.1547, 14.6464) (29.1602, 14.6475) (29.1658, 14.6485) (29.1714, 14.6496) (29.1771, 14.6507) (29.1829, 14.6519) (29.1887, 14.653) (29.1946, 14.6542) (29.2005, 14.6554) (29.2065, 14.6567) (29.2126, 14.6579) (29.2187, 14.6592) (29.2249, 14.6605) (29.2311, 14.6618) (29.2374, 14.6631) (29.2438, 14.6645) (29.2502, 14.6659) (29.2567, 14.6673) (29.2632, 14.6687) (29.2698, 14.6702) (29.2764, 14.6716) (29.2831, 14.6731) (29.2899, 14.6747) (29.2967, 14.6762) (29.3035, 14.6778) (29.3104, 14.6794) (29.3174, 14.681) (29.3244, 14.6827) (29.3314, 14.6843) (29.3386, 14.686) (29.3457, 14.6877) (29.3529, 14.6895) (29.3602, 14.6912) (29.3675, 14.693) (29.3749, 14.6948) (29.3823, 14.6967) (29.3898, 14.6985) (29.3973, 14.7004) (29.4049, 14.7023) (29.4125, 14.7043) (29.4202, 14.7062) (29.4279, 14.7082) (29.4356, 14.7102) (29.4434, 14.7123) (29.4513, 14.7143) (29.4592, 14.7164) (29.4671, 14.7185) (29.4751, 14.7207) (29.4832, 14.7228) (29.4912, 14.725) (29.4994, 14.7272) (29.5075, 14.7295) (29.5158, 14.7317) (29.524, 14.734) (29.5323, 14.7363) (29.5407, 14.7387) (29.5491, 14.741) (29.5575, 14.7434) (29.566, 14.7458) (29.5745, 14.7483) (29.583, 14.7508) (29.5917, 14.7533) (29.6003, 14.7558) (29.609, 14.7583) (29.6177, 14.7609) (29.6265, 14.7635) (29.6353, 14.7661) (29.6441, 14.7688) (29.653, 14.7714) (29.6619, 14.7741) (29.6709, 14.7769) (29.6799, 14.7796) (29.689, 14.7824) (29.6981, 14.7852) (29.7072, 14.788) (29.7163, 14.7909) (29.7255, 14.7938) (29.7348, 14.7967) (29.7441, 14.7996) (29.7534, 14.8026) (29.7627, 14.8056) (29.7721, 14.8086) (29.7815, 14.8117) (29.791, 14.8147) (29.8005, 14.8178) (29.81, 14.821) (29.8196, 14.8241) (29.8292, 14.8273) (29.8388, 14.8305) (29.8485, 14.8337) (29.8582, 14.837) (29.868, 14.8403) (29.8777, 14.8436) (29.8875, 14.8469) (29.8974, 14.8503) (29.9073, 14.8537) (29.9172, 14.8571) (29.9271, 14.8606) (29.9371, 14.864) (29.9471, 14.8675) (29.9572, 14.8711) (29.9673, 14.8746) (29.9774, 14.8782) (29.9875, 14.8818) (29.9977, 14.8855) (30.0079, 14.8891) (30.0182, 14.8928) (30.0284, 14.8965) (30.0388, 14.9003) (30.0491, 14.9041) (30.0595, 14.9079) (30.0699, 14.9117) (30.0803, 14.9156) (30.0907, 14.9194) (30.1012, 14.9234) (30.1118, 14.9273) (30.1223, 14.9313) (30.1329, 14.9353) (30.1435, 14.9393) (30.1541, 14.9433) (30.1648, 14.9474) (30.1755, 14.9515) (30.1862, 14.9557) (30.197, 14.9598) (30.2078, 14.964) (30.2186, 14.9682) (30.2294, 14.9725) (30.2403, 14.9767) (30.2512, 14.981) (30.2621, 14.9854) (30.2731, 14.9897) (30.2841, 14.9941) (30.2951, 14.9985) (30.3061, 15.003) (30.3172, 15.0074) (30.3283, 15.0119) (30.3394, 15.0165) (30.3506, 15.021) (30.3617, 15.0256) (30.3729, 15.0302) (30.3841, 15.0348) (30.3954, 15.0395) (30.4067, 15.0442) (30.418, 15.0489) (30.4293, 15.0537) (30.4407, 15.0584) (30.452, 15.0632) (30.4634, 15.0681) (30.4749, 15.0729) (30.4863, 15.0778) (30.4978, 15.0827) (30.5093, 15.0877) (30.5208, 15.0927) (30.5324, 15.0977) (30.5439, 15.1027) (30.5555, 15.1077) (30.5672, 15.1128) (30.5788, 15.1179) (30.5905, 15.1231) (30.6022, 15.1283) (30.6139, 15.1335) (30.6256, 15.1387) (30.6374, 15.1439) (30.6492, 15.1492) (30.661, 15.1545) (30.6728, 15.1599) (30.6847, 15.1653) (30.6966, 15.1707) (30.7085, 15.1761) (30.7204, 15.1815) (30.7323, 15.187) (30.7443, 15.1925) (30.7563, 15.1981) (30.7683, 15.2036) (30.7803, 15.2092) (30.7924, 15.2149) (30.8044, 15.2205) (30.8165, 15.2262) (30.8287, 15.2319) (30.8408, 15.2376) (30.853, 15.2434) (30.8627, 15.248) (30.87, 15.2515) (30.8749, 15.2539) (30.8773, 15.255) knots 0 0 0 0 0 0 0.00416667 0.00833333 0.0125 0.01666667 0.02083333 0.025 0.02916667 0.03333333 0.0375 0.04166667 0.04583333 0.05 0.05416667 0.05833333 0.0625 0.06666667 0.07083333 0.075 0.07916667 0.08333333 0.0875 0.09166667 0.09583333 0.1 0.10416667 0.10833333 0.1125 0.11666667 0.12083333 0.125 0.12916667 0.13333333 0.1375 0.14166667 0.14583333 0.15 0.15416667 0.15833333 0.1625 0.16666667 0.17083333 0.175 0.17916667 0.18333333 0.1875 0.19166667 0.19583333 0.2 0.20416667 0.20833333 0.2125 0.21666667 0.22083333 0.225 0.22916667 0.23333333 0.2375 0.24166667 0.24583333 0.25 0.25416667 0.25833333 0.2625 0.26666667 0.27083333 0.275 0.27916667 0.28333333 0.2875 0.29166667 0.29583333 0.3 0.30416667 0.30833333 0.3125 0.31666667 0.32083333 0.325 0.32916667 0.33333333 0.3375 0.34166667 0.34583333 0.35 0.35416667 0.35833333 0.3625 0.36666667 0.37083333 0.375 0.37916667 0.38333333 0.3875 0.39166667 0.39583333 0.4 0.40416667 0.40833333 0.4125 0.41666667 0.42083333 0.425 0.42916667 0.43333333 0.4375 0.44166667 0.44583333 0.45 0.45416667 0.45833333 0.4625 0.46666667 0.47083333 0.475 0.47916667 0.48333333 0.4875 0.49166667 0.49583333 0.5 0.50416667 0.50833333 0.5125 0.51666667 0.52083333 0.525 0.52916667 0.53333333 0.5375 0.54166667 0.54583333 0.55 0.55416667 0.55833333 0.5625 0.56666667 0.57083333 0.575 0.57916667 0.58333333 0.5875 0.59166667 0.59583333 0.6 0.60416667 0.60833333 0.6125 0.61666667 0.62083333 0.625 0.62916667 0.63333333 0.6375 0.64166667 0.64583333 0.65 0.65416667 0.65833333 0.6625 0.66666667 0.67083333 0.675 0.67916667 0.68333333 0.6875 0.69166667 0.69583333 0.7 0.70416667 0.70833333 0.7125 0.71666667 0.72083333 0.725 0.72916667 0.73333333 0.7375 0.74166667 0.74583333 0.75 0.75416667 0.75833333 0.7625 0.76666667 0.77083333 0.775 0.77916667 0.78333333 0.7875 0.79166667 0.79583333 0.8 0.80416667 0.80833333 0.8125 0.81666667 0.82083333 0.825 0.82916667 0.83333333 0.8375 0.84166667 0.84583333 0.85 0.85416667 0.85833333 0.8625 0.86666667 0.87083333 0.875 0.87916667 0.88333333 0.8875 0.89166667 0.89583333 0.9 0.90416667 0.90833333 0.9125 0.91666667 0.92083333 0.925 0.92916667 0.93333333 0.9375 0.94166667 0.94583333 0.95 0.95416667 0.95833333 0.9625 0.96666667 0.97083333 0.975 0.97916667 0.98333333 0.9875 0.99166667 0.99583333 1 1 1 1 1 1